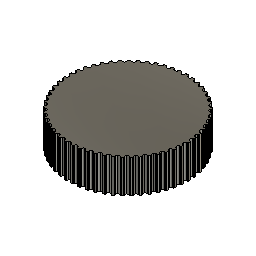
gear_57z (Autodesk Fusion 360 design; units mm, degrees)
Autodesk Fusion 360 part; units mm, degrees
sketch "Sketch1" plane through (0, 0, 0) normal (0, 0, 1) x (1, 0, 0) in component "gt2 pulley"
  circle A0 centre (0, 0) radius 18.1437 construction
  circle A1 centre (0, 0) radius 17.1397 construction
  line L0 (0, 0) -> (0, 18.1437) construction
  line L1 (0, 0) -> (0.9995, 18.1161) construction
  line L2 (0, 0) -> (1.4065, 18.0891) construction
  circle A2 centre (0, 0) radius 17.8897 construction
  arc A3 (0.3904, 17.7508) -> (0.4608, 17.4582) centre (1.3868, 17.8358) ccw
  circle A4 centre (0, 0) radius 17.7397 construction
  arc A5 (0.243, 17.888) -> (0, 17.8897) centre (0, 0) ccw
  arc A6 (0.3904, 17.7508) -> (0.243, 17.888) centre (0.241, 17.738) ccw
  arc A7 (0.4608, 17.4582) -> (0.9442, 17.1136) centre (0.9748, 17.6678) ccw
  arc A8 (0, 17.8897) -> (-0.243, 17.888) centre (0, 0) ccw
  arc A9 (-0.243, 17.888) -> (-0.3904, 17.7508) centre (-0.241, 17.738) ccw
  arc A10 (-0.4608, 17.4582) -> (-0.3904, 17.7508) centre (-1.3868, 17.8358) ccw
  arc A11 (-0.9442, 17.1136) -> (-0.4609, 17.4582) centre (-0.9748, 17.6678) ccw
  arc A12 (0.9442, 17.1136) -> (-0.9442, 17.1136) centre (0, 0) ccw
  point P0 (1.3868, 17.8358)
  point P1 (0, 17.8897)
  dimension "d18" = 36.2873
  dimension "d19" = 3.158
  dimension "d22" = 1.004
  dimension "d24" = 0.75
  dimension "d26" = 1
  dimension "d27" = 0.15
  dimension "d28" = 0.15
  dimension "d47" = 0.555
  dimension "d52" = 3.812
  constraint coincident A0.centre A1.centre
  constraint coincident A0 L0.end
  constraint vertical L0
  constraint coincident A0 L1.end
  constraint coincident A0 L2.end
  constraint concentric A1 A2
  constraint coincident A1 A7.end
  constraint coincident L1 A7.end
  constraint coincident A2 P0
  constraint coincident L2 P0
  constraint coincident P0 A3.centre
  constraint coincident A2 P1
  constraint coincident L0 P1
  constraint concentric A2 A4
  constraint coincident P1 A5.end
  constraint coincident A4 A6.centre
  constraint coincident A3.start A6.start
  constraint tangent A3 A6
  constraint tangent A3 A7
  constraint symmetric L0 A7.end A11.start
  constraint symmetric L0 A3.start A9.end
  constraint symmetric L0 A3.end A10.start
  constraint symmetric L0 A3 A10
  constraint symmetric L0 A5.start A8.end
  constraint symmetric L0 P1 A5.end
  constraint symmetric L0 A5 A8
  constraint symmetric L0 A6 A9
  constraint symmetric L0 A7 A11
  constraint coincident A1 A11.start
  constraint tangent A1 A7
  constraint coincident L1 A7.centre
  measures "d18" diameter of A0
  measures "d19" angle of L0 L1
  measures "d22" distance of A0 A1
  measures "d24" distance of A1 A2
  measures "d26" radius of A3
  measures "d27" distance of A2 A4
  measures "d28" radius of A6
  measures "d47" radius of A7
extrude "Extrude1" add sketch "Sketch1" along normal blind 10 makes body 1
pattern_circular "C-Pattern1" count 57 over 360 about axis through (0, 0, 1.75) along (0, 0, 1) of bodies 1 makes body 2 at (-1.1537, 17.1008, 3.3333) makes body 3 at (-4.4614, 16.5488, 6.6667) makes body 4 at (-4.8654, 16.4346, 3.3333) makes body 5 at (-6.6438, 15.7996, 3.3333) makes body 6 at (-8.3416, 14.9728, 3.3333) makes body 7 at (-9.9381, 13.9643, 3.3333) makes body 8 at (-11.414, 12.7863, 3.3333) makes body 9 at (-12.7513, 11.4531, 3.3333) makes body 10 at (-14.4059, 9.2865, 6.6667) makes body 11 at (-15.6105, 7.0766, 6.6667) makes body 12 at (-16.2943, 5.3164, 6.6667) makes body 13 at (-16.7802, 3.4916, 6.6667) makes body 14 at (-16.8607, 3.0796, 3.3333) makes body 15 at (-17.0972, 1.2061, 3.3333) makes body 16 at (-17.1261, -0.6821, 3.3333) makes body 17 at (-16.7133, -3.7993, 3.3333) makes body 18 at (-16.1939, -5.6149, 6.6667) makes body 19 at (-15.6536, -6.9809, 6.6667) makes body 20 at (-14.7906, -8.6606, 6.6667) makes body 21 at (-13.3628, -10.7332, 6.6667) makes body 22 at (-13.0959, -11.0573, 3.3333) makes body 23 at (-10.6923, -13.3957, 6.6667) makes body 24 at (-10.361, -13.6535, 3.3333) makes body 25 at (-8.0651, -15.1236, 6.6667) makes body 26 at (-5.7634, -16.1416, 6.6667) makes body 27 at (-3.9527, -16.6777, 6.6667) makes body 28 at (-2.094, -17.0113, 6.6667) makes body 29 at (-0.8394, -17.1191, 6.6667) makes body 30 at (0.2099, -17.1384, 3.3333) makes body 31 at (2.094, -17.0113, 3.3333) makes body 32 at (3.9527, -16.6777, 3.3333) makes body 33 at (6.5469, -15.84, 6.6667) makes body 34 at (8.2497, -15.0236, 6.6667) makes body 35 at (9.1537, -14.4906, 3.3333) makes body 36 at (10.6923, -13.3957, 3.3333) makes body 37 at (12.101, -12.1381, 3.3333) makes body 38 at (14.2329, -9.5495, 6.6667) makes body 39 at (15.197, -7.9258, 6.6667) makes body 40 at (15.7379, -6.7887, 6.6667) makes body 41 at (16.1239, -5.8128, 3.3333) makes body 42 at (16.6655, -4.0037, 3.3333) makes body 43 at (17.0048, -2.1461, 3.3333) makes body 44 at (17.1377, -0.2624, 3.3333) makes body 45 at (16.8972, 2.8729, 6.6667) makes body 46 at (16.4196, 4.9157, 6.6667) makes body 47 at (16.0144, 6.108, 6.6667) makes body 48 at (14.9472, 8.3874, 6.6667) makes body 49 at (14.7373, 8.751, 3.3333) makes body 50 at (13.5578, 10.4859, 6.6667) makes body 51 at (11.414, 12.7863, 6.6667) makes body 52 at (9.9381, 13.9643, 6.6667) makes body 53 at (8.3416, 14.9728, 6.6667) makes body 54 at (7.9723, 15.1727, 3.3333) makes body 55 at (4.8654, 16.4346, 6.6667) makes body 56 at (4.4614, 16.5488, 3.3333) makes body 57 at (1.1537, 17.1008, 6.6667)
sketch "Sketch2" plane through (0, 0, 10) normal (0, 0, 1) x (-1, 0, 0)
  arc A0 (-9.6282, -14.9178) -> (-9.5744, -15.1119) centre (-9.4942, -14.9852) ccw
  arc A1 (-9.5744, -15.1119) -> (-9.1605, -15.3664) centre (0, 0) ccw
  arc A2 (-9.1605, -15.3664) -> (-8.963, -15.3267) centre (-9.0836, -15.2376) ccw
  arc A3 (-8.7498, -15.1143) -> (-8.963, -15.3267) centre (-8.1587, -15.9209) ccw
  arc A4 (-8.1576, -15.0739) -> (-8.7498, -15.1143) centre (-8.4217, -15.562) ccw
  arc A5 (-9.7663, -14.085) -> (-8.1576, -15.0739) centre (0, 0) ccw
  arc A6 (-9.535, -14.6317) -> (-9.7663, -14.085) centre (-10.0826, -14.5411) ccw
  arc A7 (-9.6282, -14.9178) -> (-9.535, -14.6317) centre (-10.5216, -14.4685) ccw
  circle A8 centre (0, 0) radius 17.1397
  constraint coincident A1.centre A5.centre
extrude "Extrude2" add sketch "Sketch2" against normal blind 10 contours A5 A8 bodies 1 2 3 4 5 6 7 8 9 10 11 12 13 14 15 16 17 18 19 20 21 22 23 24 25 26 27 28 29 30 31 32 33 34 35 36 37 38 39 40 41 42 43 44 45 46 47 48 49 50 51 52 53 54 55 56 57
extrude "Extrude4" [suppressed] in component "gt2 pulley"
pattern_circular "C-Pattern7" [suppressed] in component "gt2 pulley"
extrude "Extrude3" [suppressed] in component "gt2 pulley"
pattern_circular "C-Pattern6" [suppressed] in component "gt2 pulley"
extrude "Extrude2'" [suppressed] in component "gt2 pulley"
pattern_circular "C-Pattern5" [suppressed] in component "gt2 pulley"
extrude "Extrude1'" [suppressed] in component "gt2 pulley"
pattern_circular "C-Pattern4" [suppressed] in component "gt2 pulley"
pattern_circular "C-Pattern3" [suppressed] in component "gt2 pulley"
pattern_circular "C-Pattern2" [suppressed] in component "gt2 pulley"
pattern_circular "C-Pattern1'" [suppressed] in component "gt2 pulley"
copy_body "Body->Comp1" [suppressed] in component "Component"
copy_body "Body->Comp2" [suppressed] in component "Component'"
copy_body "Body->Comp3" [suppressed] in component "Component''"
copy_body "Body->Comp4" [suppressed] in component "Component'''"
copy_body "Body->Comp5" [suppressed] in component "Component''''"
copy_body "Body->Comp6" [suppressed] in component "Component'''''"
copy_body "Body->Comp7" [suppressed] in component "Component''''''"
copy_body "Body->Comp8" [suppressed] in component "Component'''''''"
copy_body "Body->Comp9" [suppressed] in component "Component''''''''"
copy_body "Body->Comp10" [suppressed] in component "Component'''''''''"
copy_body "Body->Comp11" [suppressed] in component "Component''''''''''"
copy_body "Body->Comp12" [suppressed] in component "Component'''''''''''"
copy_body "Body->Comp13" [suppressed] in component "Component''''''''''''"
copy_body "Body->Comp14" [suppressed] in component "Component'''''''''''''"
copy_body "Body->Comp15" [suppressed] in component "Component''''''''''''''"
copy_body "Body->Comp16" [suppressed] in component "Component'''''''''''''''"
copy_body "Body->Comp17" [suppressed] in component "Component''''''''''''''''"
copy_body "Body->Comp18" [suppressed] in component "Component'''''''''''''''''"
copy_body "Body->Comp19" [suppressed] in component "Component''''''''''''''''''"
copy_body "Body->Comp20" [suppressed] in component "Component'''''''''''''''''''"
component "gt2 pulley" placed x (1, 0, 0) y (0, 1, 0) z (0, 0, 1) at (0, 0, 0)
equation "NumTeeth = 57" comment "min 20"
equation "ToothPitch = 2 mm"
equation "PullyDia = NumTeeth * ToothPitch / PI"
equation "ToothAng = ( ( 360 / NumTeeth ) * 1 deg )"
equation "TransOffsetAngle = ToothAng * 0.2"
equation "Sholulder_Radius = 0.15 mm"
equation "Root_Radius = 0.555 mm"
equation "TransRadius = 1 mm"
equation "ToolHeight = 0.75 mm"
equation "PLD = 0.254 mm"
equation "d18 = PullyDia"
equation "d19 = ToothAng / 2"
equation "d22 = PLD + ToolHeight"
equation "d24 = ToolHeight"
equation "d26 = TransRadius"
equation "d27 = Sholulder_Radius"
equation "d31 = NumTeeth"
equation "d33 = NumTeeth"
equation "d35 = NumTeeth"
equation "d37 = NumTeeth"
equation "d41 = NumTeeth"
equation "d45 = NumTeeth"
equation "d47 = Root_Radius"
equation "d50 = NumTeeth"
